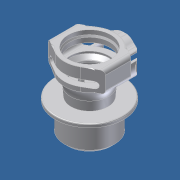
# Autodesk Inventor part: HFC12_bodyY
Saved by Autodesk Inventor 2012 SP1 (Build 160190100, 190)
## iProperties
Category: PARTsolutions
Created: 2012-06-06
Part Number: HFC12_bodyY
Catalog Web Link: www.cadenas.de
Description: HFC12 BODY - HFC12 BODY
Document SubType Name: Modeling
Designer: PARTsolutions
Material: Default
Mass: 19.9352 g
Surface Area: 116.481 cm^2
Volume: 19.9352 cm^3
Density: 1 g/cm^3
NB: HFC12_bodyY
NN: HFC12 BODY
NT: HFC12 BODY
NBSYN: $PN.$VN.$PANELMOUNT.
LINA: HFC12_bodyY
PN: HFC12_body
PANELMOUNT: Y
KT: DUMMY
SUPPLIER: Colder
ARTICLENO: HFC12_bodyYHI
BOMINFO: HFC12_bodyY
CREATOR: CADENAS GmbH
PSOL_IDENT_0: {\\10.0.0.251\data_v9\23d-libs\colder\single_line\3_8_nom_flow\hfc12_series\bodies\parts\hfc12_body.
PSOL_IDENT_1: prj},181 {VTYP=3D},{NB=HFC12_bodyY},{LINA=HFC12_bodyY},{NN=HFC12 BODY},{DATE=12.11.2009 06:46:58},{G
PSOL_IDENT_2: EOMDATE=12.11.2009 06:46:00},{VERSION=},{LINEID=10},{LINESUBID=-1},{WBVAR=VN,PANELMOUNT}  {NB=HFC12_
PSOL_IDENT_3: bodyY},{LINA=HFC12_bodyY},{KT=DUMMY},{PN=HFC12_body},{VN=},{PANELMOUNT=Y}
Title: HFC12_bodyY
Author: Cadenas PARTsolutions
Comments: HFC12 BODY
Autodesk Inventor part; units mm, degrees
sketch "Sketch1" plane through (0, 0, 0) normal (0, 1, 0) x (-1, 0, 0)
  arc A0 (17.272, 42.926) -> (14.986, 45.212) centre (14.986, 42.926) ccw
  line L0 (14.986, 45.212) -> (-14.986, 45.212)
  arc A1 (-14.986, 45.212) -> (-17.272, 42.926) centre (-14.986, 42.926) ccw
  line L1 (-17.272, 42.926) -> (-17.272, 34.8353)
  arc A2 (-17.272, 34.8353) -> (-16.2172, 32.9103) centre (-14.986, 34.8364) ccw
  line L2 (-16.2172, 32.9103) -> (16.2172, 32.9103)
  arc A3 (16.2172, 32.9103) -> (17.272, 34.8353) centre (14.986, 34.8364) ccw
  line L3 (17.272, 34.8353) -> (17.272, 42.926)
  constraints: 8 end point, 8 point on circle, 4 centre point
extrude "Extrusion1" add sketch "Sketch1" along normal mid plane 20
sketch "Sketch4" plane through (0, 0, 0) normal (0, 1, 0) x (-1, 0, 0)
  line L0 (0, 0) -> (0, 45.212)
  arc A0 (17.272, 42.926) -> (14.986, 45.212) centre (14.986, 42.926) ccw
  line L1 (14.986, 45.212) -> (12.827, 45.212)
  line L2 (12.827, 45.212) -> (12.827, 42.672)
  line L3 (12.827, 42.672) -> (12.2555, 41.6821)
  line L4 (12.2555, 41.6821) -> (12.2555, 38.862)
  line L5 (12.2555, 38.862) -> (12.9159, 38.862)
  arc A1 (12.9159, 34.8488) -> (12.9159, 38.862) centre (12.9159, 36.8554) ccw
  line L6 (12.9159, 34.8488) -> (11.684, 34.8488)
  line L7 (11.684, 34.8488) -> (11.684, 33.6804)
  line L8 (11.684, 33.6804) -> (9.6684, 31.6648)
  arc A2 (9.6684, 31.6648) -> (9.2964, 30.7667) centre (10.5664, 30.7667) ccw
  line L9 (9.2964, 30.7667) -> (9.2964, 22.5298)
  arc A3 (8.5344, 21.7678) -> (9.2964, 22.5298) centre (8.5344, 22.5298) ccw
  line L10 (8.5344, 21.7678) -> (8.3811, 16.1798)
  arc A4 (8.382, 16.1036) -> (8.3811, 16.1798) centre (5.08, 16.1036) ccw
  line L11 (8.382, 16.1036) -> (8.382, 0)
  line L12 (8.382, 0) -> (12.7, 0)
  arc A5 (12.7, 0) -> (11.557, 4.6818) centre (2.54, 0) ccw
  arc A6 (10.442, 10.1175) -> (11.557, 4.6818) centre (20.574, 9.3636) ccw
  line L13 (10.442, 10.1175) -> (11.557, 25.1035)
  arc A7 (16.2172, 32.9103) -> (11.557, 25.1035) centre (21.689, 24.3496) ccw
  arc A8 (16.2172, 32.9103) -> (17.272, 34.8353) centre (14.986, 34.8364) ccw
  line L14 (17.272, 34.8353) -> (17.272, 42.926)
  constraints: 30 end point, 18 point on circle, 9 centre point
revolve "Revolution1" add sketch "Sketch4" angle 360 about axis through (0, 0, 0) along (0, 0, -1)
sketch "Sketch7" plane through (0, 0, 45.212) normal (0, 0, 1) x (1, 0, 0)
  line L0 (-44.1604, 28.5772) -> (-44.1604, -35.0676)
  line L1 (-44.1604, -35.0676) -> (41.3415, -35.0676)
  line L2 (41.3415, -35.0676) -> (41.3415, 28.5772)
  line L3 (41.3415, 28.5772) -> (-44.1604, 28.5772)
  line L4 (-17.272, 7.6256) -> (-17.272, -7.6256)
  line L5 (-17.272, -7.6256) -> (-7.62, -13.1982)
  arc A0 (-7.62, -13.1982) -> (7.62, -13.1982) centre (0, 0) ccw
  line L6 (7.62, -13.1982) -> (17.272, -7.6256)
  line L7 (17.272, -7.6256) -> (17.272, 7.6256)
  line L8 (17.272, 7.6256) -> (7.62, 13.1982)
  arc A1 (7.62, 13.1982) -> (-7.62, 13.1982) centre (0, 0) ccw
  line L9 (-7.62, 13.1982) -> (-17.272, 7.6256)
  constraints: 20 end point, 4 point on circle, 2 centre point
extrude "Extrusion2" cut sketch "Sketch7" against normal blind 23.622
sketch "Sketch10" plane through (0, 17, 0) normal (0, 1, 0) x (-1, 0, 0)
  arc A0 (-10.9459, 34.8488) -> (-1.27, 21.59) centre (-1.27, 31.75) ccw
  line L0 (-1.27, 21.59) -> (1.27, 21.59)
  arc A1 (1.27, 21.59) -> (10.9459, 34.8488) centre (1.27, 31.75) ccw
  line L1 (10.9459, 34.8488) -> (9.6024, 34.8488)
  arc A2 (1.27, 22.86) -> (9.6024, 34.8488) centre (1.27, 31.75) ccw
  line L2 (1.27, 22.86) -> (-1.27, 22.86)
  arc A3 (-9.6024, 34.8488) -> (-1.27, 22.86) centre (-1.27, 31.75) ccw
  line L3 (-9.6024, 34.8488) -> (-10.9459, 34.8488)
  constraints: 8 end point, 8 point on circle, 4 centre point
extrude "Extrusion3" add sketch "Sketch10" along normal mid plane 20
sketch "Sketch13" plane through (0, 17, 0) normal (0, 1, 0) x (-1, 0, 0)
  arc A0 (10.6428, 38.862) -> (10.6428, 40.1117) centre (10.6428, 39.4869) ccw
  line L0 (10.6428, 40.1117) -> (8.763, 40.1117)
  arc A1 (7.3853, 40.263) -> (8.763, 40.1117) centre (8.763, 46.4617) ccw
  arc A2 (7.302, 40.2821) -> (7.3853, 40.263) centre (8.8662, 46.9259) ccw
  arc A3 (5.7906, 40.8707) -> (7.302, 40.2821) centre (8.6324, 45.933) ccw
  arc A4 (5.7906, 40.8707) -> (1.3993, 42.1353) centre (0.9081, 32.173) ccw
  arc A5 (1.3993, 42.1353) -> (1.1765, 42.1436) centre (0.9318, 32.6554) ccw
  arc A6 (1.1765, 42.1436) -> (-1.1794, 42.1436) centre (-0.0014, -3.5453) ccw
  arc A7 (-1.1794, 42.1436) -> (-1.4021, 42.1353) centre (-0.9347, 32.6554) ccw
  arc A8 (-1.4021, 42.1353) -> (-5.7936, 40.8706) centre (-0.9109, 32.1731) ccw
  arc A9 (-7.3049, 40.2821) -> (-5.7936, 40.8706) centre (-8.6344, 45.9308) ccw
  arc A10 (-8.4713, 40.112) -> (-7.3049, 40.2821) centre (-8.8697, 46.9302) ccw
  arc A11 (-8.763, 40.1117) -> (-8.4713, 40.112) centre (-8.6232, 46.4602) ccw
  line L1 (-8.763, 40.1117) -> (-10.6428, 40.1117)
  arc A12 (-10.6428, 40.1117) -> (-10.6428, 38.862) centre (-10.6428, 39.4869) ccw
  line L2 (-10.6428, 38.862) -> (-6.604, 38.862)
  arc A13 (-1.27, 40.64) -> (-6.604, 38.862) centre (-1.27, 31.75) ccw
  line L3 (-1.27, 40.64) -> (1.27, 40.64)
  arc A14 (6.604, 38.862) -> (1.27, 40.64) centre (1.27, 31.75) ccw
  line L4 (6.604, 38.862) -> (10.6428, 38.862)
  constraints: 30 point on circle, 15 centre point, 10 end point
extrude "Extrusion4" add sketch "Sketch13" along normal mid plane 20
sketch "Sketch16" plane through (0, 0, 45.212) normal (0, 0, 1) x (1, 0, 0)
  arc A0 (-13.3063, 13.3209) -> (-12.3271, 13.1781) centre (-12.8063, 13.3209) ccw
  line L0 (-12.3271, 13.1781) -> (-11.2512, 16.7871)
  arc A1 (-9.3406, 19.0438) -> (-11.2512, 16.7871) centre (-7.7197, 15.7343) ccw
  arc A2 (9.3406, 19.0438) -> (-9.3406, 19.0438) centre (0, -0.0275) ccw
  arc A3 (11.2512, 16.7871) -> (9.3406, 19.0438) centre (7.7197, 15.7343) ccw
  line L1 (11.2512, 16.7871) -> (12.3271, 13.1781)
  arc A4 (12.3271, 13.1781) -> (13.3063, 13.3209) centre (12.8063, 13.3209) ccw
  line L2 (13.3063, 13.3209) -> (13.3063, 33.1138)
  line L3 (13.3063, 33.1138) -> (-13.3063, 33.1138)
  line L4 (-13.3063, 33.1138) -> (-13.3063, 13.3209)
  constraints: 10 end point, 10 point on circle, 5 centre point
extrude "Extrusion5" cut sketch "Sketch16" against normal blind 23.622
sketch "Sketch_5" plane through (0, 0, 0) normal (0, 1, 0) x (-1, 0, 0)
  arc A0 (12.9159, 34.8387) -> (12.9159, 38.8719) centre (12.9059, 36.8553) ccw
  line L0 (12.9159, 38.8719) -> (-12.9159, 38.8719)
  arc A1 (-12.9159, 38.8719) -> (-12.9159, 34.8387) centre (-12.9059, 36.8553) ccw
  line L1 (-12.9159, 34.8387) -> (12.9159, 34.8387)
  constraints: 4 end point, 4 point on circle, 2 centre point
extrude "Extrusion6" cut sketch "Sketch_5" along normal mid plane 30.48
sketch "Sketch22" plane through (0, 0, 0) normal (0, 1, 0) x (-1, 0, 0)
  line L0 (0, 0) -> (0, 45.212)
  line L1 (0, 45.212) -> (12.827, 45.212)
  line L2 (12.827, 45.212) -> (12.827, 42.672)
  line L3 (12.827, 42.672) -> (12.2555, 41.6821)
  line L4 (12.2555, 41.6821) -> (12.2555, 38.862)
  line L5 (12.2555, 38.862) -> (12.9159, 38.862)
  arc A0 (12.9159, 34.8488) -> (12.9159, 38.862) centre (12.9159, 36.8554) ccw
  line L6 (12.9159, 34.8488) -> (11.684, 34.8488)
  line L7 (11.684, 34.8488) -> (11.684, 33.6804)
  line L8 (11.684, 33.6804) -> (9.6684, 31.6648)
  arc A1 (9.6684, 31.6648) -> (9.2964, 30.7667) centre (10.5664, 30.7667) ccw
  line L9 (9.2964, 30.7667) -> (9.2964, 22.5298)
  arc A2 (8.5344, 21.7678) -> (9.2964, 22.5298) centre (8.5344, 22.5298) ccw
  line L10 (8.5344, 21.7678) -> (8.3811, 16.1798)
  arc A3 (8.382, 16.1036) -> (8.3811, 16.1798) centre (5.08, 16.1036) ccw
  line L11 (8.382, 16.1036) -> (8.382, 0)
  line L12 (8.382, 0) -> (0, 0)
  line L13 (0, 0) -> (0, 45.212)
  constraints: 28 end point, 8 point on circle, 4 centre point
revolve "Revolution2" cut sketch "Sketch22" angle 360 about axis through (0, 0, 0) along (0, 0, -1)
sketch "Sketch_2" plane through (0, 0, 21.7678) normal (0, 0, 1) x (1, 0, 0)
  circle A0 centre (0, 0) radius 9.296
  arc A1 (0.889, -4.6887) -> (1.2032, -4.9355) centre (1.143, -4.6887) ccw
  arc A2 (1.2032, -4.9355) -> (4.9355, -1.2032) centre (0, 0) ccw
  arc A3 (4.9355, -1.2032) -> (4.6887, -0.889) centre (4.6887, -1.143) ccw
  line L0 (4.6887, -0.889) -> (2.1251, -0.889)
  arc A4 (2.1251, -0.889) -> (1.9014, -1.0227) centre (2.1251, -1.143) ccw
  arc A5 (1.0227, -1.9014) -> (1.9014, -1.0227) centre (0, 0) ccw
  arc A6 (1.0227, -1.9014) -> (0.889, -2.1251) centre (1.143, -2.1251) ccw
  line L1 (0.889, -2.1251) -> (0.889, -4.6887)
  arc A7 (0.889, 2.1251) -> (1.0227, 1.9014) centre (1.143, 2.1251) ccw
  arc A8 (1.9014, 1.0227) -> (1.0227, 1.9014) centre (0, 0) ccw
  arc A9 (1.9014, 1.0227) -> (2.1251, 0.889) centre (2.1251, 1.143) ccw
  line L2 (2.1251, 0.889) -> (4.6887, 0.889)
  arc A10 (4.6887, 0.889) -> (4.9355, 1.2032) centre (4.6887, 1.143) ccw
  arc A11 (4.9355, 1.2032) -> (1.2032, 4.9355) centre (0, 0) ccw
  arc A12 (1.2032, 4.9355) -> (0.889, 4.6887) centre (1.143, 4.6887) ccw
  line L3 (0.889, 4.6887) -> (0.889, 2.1251)
  arc A13 (-4.6887, -0.889) -> (-4.9355, -1.2032) centre (-4.6887, -1.143) ccw
  arc A14 (-4.9355, -1.2032) -> (-1.2032, -4.9355) centre (0, 0) ccw
  arc A15 (-1.2032, -4.9355) -> (-0.889, -4.6887) centre (-1.143, -4.6887) ccw
  line L4 (-0.889, -4.6887) -> (-0.889, -2.1251)
  arc A16 (-0.889, -2.1251) -> (-1.0227, -1.9014) centre (-1.143, -2.1251) ccw
  arc A17 (-1.9014, -1.0227) -> (-1.0227, -1.9014) centre (0, 0) ccw
  arc A18 (-1.9014, -1.0227) -> (-2.1251, -0.889) centre (-2.1251, -1.143) ccw
  line L5 (-2.1251, -0.889) -> (-4.6887, -0.889)
  arc A19 (-4.9355, 1.2032) -> (-4.6887, 0.889) centre (-4.6887, 1.143) ccw
  line L6 (-4.6887, 0.889) -> (-2.1251, 0.889)
  arc A20 (-2.1251, 0.889) -> (-1.9014, 1.0227) centre (-2.1251, 1.143) ccw
  arc A21 (-1.0227, 1.9014) -> (-1.9014, 1.0227) centre (0, 0) ccw
  arc A22 (-1.0227, 1.9014) -> (-0.889, 2.1251) centre (-1.143, 2.1251) ccw
  line L7 (-0.889, 2.1251) -> (-0.889, 4.6887)
  arc A23 (-0.889, 4.6887) -> (-1.2032, 4.9355) centre (-1.143, 4.6887) ccw
  arc A24 (-1.2032, 4.9355) -> (-4.9355, 1.2032) centre (0, 0) ccw
  constraints: 48 point on circle, 25 centre point, 16 end point
extrude "Extrusion7" add sketch "Sketch_2" along normal mid plane 11.176
sketch "Sketch_4" plane through (0, 0, 0) normal (1, 0, 0) x (0, 1, 0)
  line L0 (0, 16.1798) -> (0, 19.558)
  line L1 (-20.1295, 19.558) -> (-6.604, 19.558)
  arc A0 (-6.8272, 19.0261) -> (-6.604, 19.558) centre (-7.366, 19.565) ccw
  line L2 (-6.8272, 19.0261) -> (-7.4149, 18.4385)
  arc A1 (-7.4149, 18.4385) -> (-8.3816, 16.1544) centre (-5.08, 16.1036) ccw
  line L3 (-8.3816, 16.1544) -> (-8.3816, 0)
  line L4 (-8.3816, 0) -> (-13.1915, 0)
  line L5 (-13.1915, 0) -> (-15.0813, 1.8898)
  line L6 (-15.0813, 1.8898) -> (-15.0813, 16.6658)
  arc A2 (-15.0813, 16.6658) -> (-15.8369, 17.526) centre (-15.8369, 16.764) ccw
  line L7 (-15.8369, 17.526) -> (-20.6375, 17.526)
  line L8 (-20.6375, 17.526) -> (-20.6375, 19.05)
  arc A3 (-20.1295, 19.558) -> (-20.6375, 19.05) centre (-20.1295, 19.05) ccw
  constraints: 18 end point, 8 point on circle, 4 centre point
revolve "Revolution3" add sketch "Sketch_4" angle 360 about axis through (0, 0, 16.1798) along (0, 0, 1)
ref_plane "0_XY" through (0, 0, 0) normal (0, 0, 1) x (1, 0, 0)
ref_plane "0_YZ" through (0, 0, 0) normal (1, 0, 0) x (0, 1, 0)
ref_plane "0_ZX" through (0, 0, 0) normal (0, 1, 0) x (0, 0, 1)
body "Solid1"
